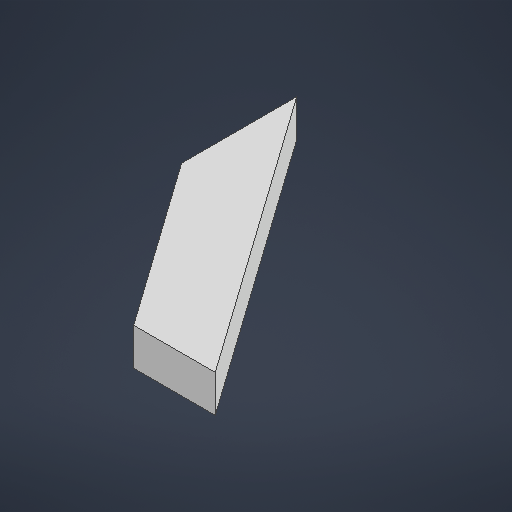
# Autodesk Inventor part: S_2x4x14.71
Saved by Autodesk Inventor 2027.1 (Build 311270010, 270A)
## iProperties
Created: 2026-09-01
Part Number: S_2x4x14.71
Material: Generic
Document SubType Name: Modeling
Designer: jorda
Density: 1 g/cm^3
Appearance: Default
Author: jorda
Autodesk Inventor part; units mm, degrees
ref_plane "YZ Plane" through (0, 0, 0) normal (1, 0, 0) x (0, 1, 0)
ref_plane "XZ Plane" through (0, 0, 0) normal (0, 1, 0) x (-1, 0, 0)
ref_plane "XY Plane" through (0, 0, 0) normal (0, 0, 1) x (1, 0, 0)
sketch "Sketch1" plane through (0, 0, 0) normal (0, 1, 0) x (-1, 0, 0)
  line L0 (0, 0) -> (83.5957, 0)
  line L1 (0, 0) -> (202.8769, -286.4145)
  line L2 (202.8769, -168.3971) -> (202.8769, -286.4145)
  line L3 (202.8769, -168.3971) -> (83.5957, 0)
  constraints: 8 end point, 1 horizontal, 1 vertical
extrude "Extrusion1" add sketch "Sketch1" along normal blind 38.1
body "Solid1"
